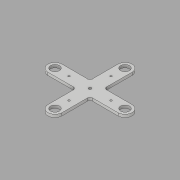
# Autodesk Inventor part: e_support 1
Saved by Autodesk Inventor 2019 (Build 230136000, 136)
## iProperties
Created: 2021-11-01
Part Number: e_support 1
Material: Generic
Document SubType Name: Modeling
Designer: Mohamed
Density: 1 g/cm^3
Appearance: Default
Author: Mohamed
Autodesk Inventor part; units mm, degrees
ref_plane "YZ Plane" through (0, 0, 0) normal (1, 0, 0) x (0, 1, 0)
ref_plane "XZ Plane" through (0, 0, 0) normal (0, 1, 0) x (-1, 0, 0)
ref_plane "XY Plane" through (0, 0, 0) normal (0, 0, 1) x (1, 0, 0)
sketch "Sketch1" plane through (0, 0, 0) normal (0, 1, 0) x (-1, 0, 0)
  circle A0 centre (75, -75) radius 9.5
  arc A1 (75, -90) -> (75, -60) centre (75, -75) ccw
  circle A2 centre (0, 0) radius 9.5
  arc A3 (15, 0) -> (-15, 0) centre (0, 0) ccw
  circle A4 centre (-75, -75) radius 9.5
  arc A5 (-75, -60) -> (-75, -90) centre (-75, -75) ccw
  circle A6 centre (0, -150) radius 9.5
  arc A7 (-15, -150) -> (15, -150) centre (0, -150) ccw
  line L0 (-75, -60) -> (-20, -60)
  line L1 (-75, -90) -> (-20, -90)
  line L2 (75, -60) -> (20, -60)
  line L3 (75, -90) -> (20, -90)
  line L4 (15, 0) -> (15, -55)
  line L5 (15, -95) -> (15, -150)
  line L6 (-15, 0) -> (-15, -55)
  line L7 (-15, -95) -> (-15, -150)
  arc A8 (15, -55) -> (20, -60) centre (20, -55) ccw
  arc A9 (-20, -60) -> (-15, -55) centre (-20, -55) ccw
  arc A10 (20, -90) -> (15, -95) centre (20, -95) ccw
  arc A11 (-15, -95) -> (-20, -90) centre (-20, -95) ccw
  circle A12 centre (0, -30) radius 2
  circle A13 centre (0, -120) radius 2
  circle A14 centre (-45, -75) radius 2
  circle A15 centre (45, -75) radius 2
  circle A16 centre (0, -75) radius 3
  point P0 (15, -60)
  point P1 (15, -90)
  dimension "d5" = 19
  dimension "d6" = 30
  dimension "d7" = 19
  dimension "d8" = 30
  dimension "d9" = 19
  dimension "d10" = 30
  dimension "d11" = 19
  dimension "d12" = 30
  dimension "d13" = 5
  dimension "d15" = 4
  dimension "d17" = 4
  dimension "d19" = 4
  dimension "d21" = 4
  dimension "d22" = 6
  constraints: 17 centre point, 16 end point, 16 point on circle, 14 tangent, 8 point on line, 4 coincident, 4 perpendicular, 3 equal radius
  measures "d5" diameter of A0
  measures "d6" diameter of A1
  measures "d7" diameter of A2
  measures "d8" diameter of A3
  measures "d9" diameter of A4
  measures "d10" diameter of A5
  measures "d11" diameter of A6
  measures "d12" diameter of A7
  measures "d13" radius of A8
  measures "d15" diameter of A12
  measures "d17" diameter of A13
  measures "d19" diameter of A14
  measures "d21" diameter of A15
  measures "d22" diameter of A16
extrude "Extrusion1" add sketch "Sketch1" along normal blind 6
body "Solid1"
